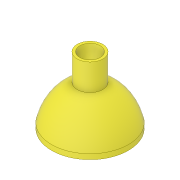
# Autodesk Inventor part: nozzle
Saved by Autodesk Inventor 2018 (Build 220112000, 112)
## iProperties
Created: 2017-11-20
Part Number: nozzle
Material: PVC-Piping
Document SubType Name: Modeling
Designer: Udara Wanasinghe
Density: 1.4 g/cm^3
Appearance: Smooth - White(1)
Mass: 0.633207 g
Surface Area: 11.0633 cm^2
Volume: 0.452291 cm^3
Author: Udara Wanasinghe
Autodesk Inventor part; units mm, degrees
ref_plane "YZ Plane" through (0, 0, 0) normal (1, 0, 0) x (0, 1, 0)
sketch "Sketch1" plane through (0, 0, 0) normal (0, 1, 0) x (-1, 0, 0)
  circle A0 centre (0, 0) radius 7.5
  dimension "d0" = 15
  constraints: 1 centre point, 1 coincident
  measures "d0" diameter of A0
extrude "Extrusion1" add sketch "Sketch1" along normal blind 1
hole "Hole1" at (0, 1, 0) direction (0, -1, 0) diameter 1 end through all
pattern_linear "Rectangular Pattern1" count 7 spacing 1.8 along (0, 0, 1) of "Hole1" first direction both ways yes
pattern_circular "Circular Pattern1" count 10 over 360 about axis through (0, -10, 0) along (0, 1, 0) of "Hole1", "Rectangular Pattern1"
ref_plane "Work Plane1" through (0, 0, 0) normal (-1, 0, 0) x (0, 0, 1)
sketch "Sketch3" plane through (0, 0, 0) normal (-1, 0, 0) x (0, 0, 1)
  line L0 (7.5, 1) -> (-7.5, 1) projected
  arc A0 (0, 8.8133) -> (-7.5, 1) centre (2.4662, -1.0603) ccw
  arc A1 (0, 7.8133) -> (-6.5103, 1) centre (2.4662, -1.0603) ccw
  line L1 (0, 1) -> (0, 9.7255) construction
  line L2 (0, 8.8133) -> (0, 7.8133)
  line L3 (-7.5, 1) -> (-6.5103, 1)
  line L4 (0, -3.2511) -> (0, 12.0847) projected
  point P0 (0, 0)
  dimension "d19" = 1
  constraints: 6 end point, 4 point on circle, 2 centre point, 2 collinear, 2 point on line, 1 concentric, 1 midpoint, 1 vertical
  measures "d19" distance of L2.start L2.end
revolve "Revolution1" add sketch "Sketch3" angle 360 about axis through (0, -10, 0) along (0, 1, 0) contours L0 A0 L2 A1
ref_plane "Work Plane2" through (0, 8, 0) normal (0, 1, 0) x (1, 0, 0)
sketch "Sketch4" plane through (0, 8, 0) normal (0, 1, 0) x (1, 0, 0)
  circle A0 centre (0, 0) radius 1.5
  dimension "d22" = 3
  constraints: 1 centre point, 1 coincident
  measures "d22" diameter of A0
extrude "Extrusion2" cut sketch "Sketch4" along normal mid plane 4
sketch "Sketch5" plane through (0, 8, 0) normal (0, 1, 0) x (1, 0, 0)
  circle A0 centre (0, 0) radius 2.5
  circle A1 centre (0, 0) radius 2
  dimension "d25" = 5
  dimension "d26" = 4
  constraints: 2 centre point, 2 coincident
  measures "d25" diameter of A0
  measures "d26" diameter of A1
extrude "Extrusion3" add sketch "Sketch5" along normal blind 5 and the other way blind 0.5
body "Solid1"
